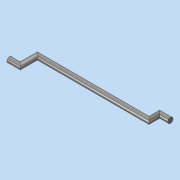
# Autodesk Inventor part: foreDivePlanesLinkage
Saved by Autodesk Inventor 2017 (Build 210142000, 142)
## iProperties
Created: 2016-12-10
Part Number: foreDivePlanesLinkage
Material: Stainless Steel
Document SubType Name: Modeling
Designer: techn
Density: 8 g/cm^3
Appearance: Semi-Polished
Mass: 0.735813 g
Surface Area: 2.33963 cm^2
Volume: 0.0919766 cm^3
Author: techn
Autodesk Inventor part; units mm, degrees
ref_plane "XZ Plane" through (0, 0, 0) normal (0, 1, 0) x (-1, 0, 0)
ref_plane "XY Plane" through (0, 0, 0) normal (0, 0, 1) x (1, 0, 0)
sketch "Sketch1" plane through (0, 0, 0) normal (0, 1, 0) x (-1, 0, 0)
  line L0 (-33.0454, 0) -> (0, 0)
  line L1 (0, 0) -> (0, 5.08)
  line L2 (0, 5.08) -> (3.175, 5.08)
  line L3 (-33.0454, 0) -> (-33.0454, -3.175)
  line L4 (-33.0454, -3.175) -> (-36.2204, -3.175)
  dimension "d1" = 33.0454
  dimension "d6" = 5.08
  dimension "d7" = 3.175
  dimension "d8" = 3.175
  dimension "d9" = 3.175
  constraints: 10 end point, 2 perpendicular, 2 vertical, 1 horizontal
  measures "d1" distance of L0.start L0.end
  measures "d6" distance of L0.end L1.end
  measures "d7" distance of L1.end L2.end
  measures "d8" distance of L0.start L3.end
  measures "d9" distance of L3.end L4.end
ref_plane "Work Plane1" through (36.2204, 0, -3.175) normal (1, 0, 0) x (0, 1, 0)
sketch "Sketch2" plane through (36.2204, 0, -3.175) normal (1, 0, 0) x (0, 1, 0)
  circle A0 centre (0, 0) radius 0.8
  point P0 (0, 3.175)
  dimension "d10" = 1.6
  constraints: 1 centre point
  measures "d10" diameter of A0
sweep "Sweep1" add profiles "Sketch2" path "Sketch1"
body "Solid1"
